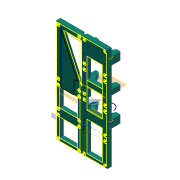
# Autodesk Inventor part: 30_CUBE_openSIM_base_v3
Saved by Autodesk Inventor 2019 (Build 230136000, 136)
## iProperties
Created: 2019-07-01
Part Number: 30_CUBE_openSIM_base_v3
Material: Generic
Document SubType Name: Modeling
Designer: diederichbenedict
Density: 1 g/cm^3
Appearance: IPHT_Türkis
Author: diederichbenedict
Autodesk Inventor part; units mm, degrees
ref_plane "YZ Plane" through (0, 0, 0) normal (1, 0, 0) x (0, 1, 0)
ref_plane "XZ Plane" through (0, 0, 0) normal (0, 1, 0) x (-1, 0, 0)
ref_plane "Work Plane1" through (181.6, 41.8, 16) normal (0, 0, -1) x (-1, 0, 0)
sketch "Sketch1" plane through (0, 41.8, 0) normal (0, 0, 1) x (1, 0, 0)
  circle A0 centre (0.9, -0.9) radius 1.45 construction
  line L0 (4, -1.5) -> (1.5, -4) construction
  line L1 (4, -1.5) -> (4, 4) construction
  line L2 (4, 4) -> (-2, 4) construction
  arc A1 (-2, 4) -> (-4, 2) centre (-2, 2) ccw construction
  line L3 (-4, 2) -> (-4, -4) construction
  line L4 (-4, -4) -> (1.5, -4) construction
  arc A2 (45.8, 2) -> (43.8, 4) centre (43.8, 2) ccw construction
  line L5 (43.8, 4) -> (37.8, 4) construction
  line L6 (37.8, 4) -> (37.8, -1.5) construction
  line L7 (40.3, -4) -> (45.8, -4) construction
  line L8 (45.8, -4) -> (45.8, 2) construction
  circle A3 centre (40.9, -0.9) radius 1.45 construction
  line L9 (37.8, -40.3) -> (40.3, -37.8) construction
  line L10 (37.8, -40.3) -> (37.8, -45.8) construction
  line L11 (37.8, -45.8) -> (43.8, -45.8) construction
  arc A4 (43.8, -45.8) -> (45.8, -43.8) centre (43.8, -43.8) ccw construction
  line L12 (45.8, -43.8) -> (45.8, -37.8) construction
  line L13 (45.8, -37.8) -> (40.3, -37.8) construction
  circle A5 centre (40.9, -40.9) radius 1.45 construction
  circle A6 centre (0.9, -40.9) radius 1.45 construction
  line L14 (1.5, -37.8) -> (4, -40.3) construction
  line L15 (1.5, -37.8) -> (-4, -37.8) construction
  line L16 (-4, -37.8) -> (-4, -43.8) construction
  arc A7 (-4, -43.8) -> (-2, -45.8) centre (-2, -43.8) ccw construction
  line L17 (-2, -45.8) -> (4, -45.8) construction
  line L18 (4, -45.8) -> (4, -40.3) construction
  line L19 (40.3, -4) -> (37.8, -1.5) construction
  line L20 (-2, 154) -> (93.8, 154)
  line L21 (95.8, 152) -> (95.8, -43.8)
  line L22 (93.8, -45.8) -> (-2, -45.8)
  line L23 (-4, -43.8) -> (-4, 152)
  line L24 (90.3, -37.8) -> (90.3, 146)
  line L25 (87.8, 148.5) -> (4, 148.5)
  line L26 (1.5, 146) -> (1.5, -37.8)
  line L27 (4, -40.3) -> (87.8, -40.3)
  line L28 (87.8, -40.3) -> (90.3, -37.8)
  line L29 (4, -40.3) -> (1.5, -37.8)
  line L30 (4, 148.5) -> (1.5, 146)
  line L31 (90.3, 146) -> (87.8, 148.5)
  arc A8 (95.8, 152) -> (93.8, 154) centre (93.8, 152) ccw
  arc A9 (93.8, -45.8) -> (95.8, -43.8) centre (93.8, -43.8) ccw
  arc A10 (-4, -43.8) -> (-2, -45.8) centre (-2, -43.8) ccw
  arc A11 (-2, 154) -> (-4, 152) centre (-2, 152) ccw
  circle A12 centre (1, -1) radius 1.4
  circle A13 centre (40.8, -1) radius 1.4
  circle A14 centre (90.8, -40.8) radius 1.4
  circle A15 centre (1, -40.8) radius 1.4
  circle A16 centre (45.9, 104.1) radius 44.4 construction
  line L32 (45.8, -37.8) -> (87.8, -37.8)
  line L33 (87.8, -37.8) -> (87.8, 146)
  line L34 (45.9, 148.5) -> (45.9, -40.3)
  line L35 (87.8, 146) -> (45.9, 146)
  line L36 (77.4, 111.7) -> (64.2, 111.7) construction
  line L37 (64.2, 96.7) -> (77.4, 96.7) construction
  line L38 (77.4, 61.7) -> (64.2, 61.7) construction
  line L39 (64.2, 46.7) -> (77.4, 46.7) construction
  line L40 (45.9, 111.7) -> (87.8, 111.7)
  line L41 (87.8, 111.7) -> (87.8, 96.7)
  line L42 (87.8, 96.7) -> (45.9, 96.7)
  line L43 (45.9, 96.7) -> (45.9, 111.7)
  line L44 (45.9, 61.7) -> (87.8, 61.7)
  line L45 (87.8, 61.7) -> (87.8, 46.7)
  line L46 (87.8, 46.7) -> (45.9, 46.7)
  line L47 (45.9, 46.7) -> (45.9, 61.7)
  point P0 (95.8, -45.8)
  point P1 (95.8, 154)
  point P2 (-4, -45.8)
  point P3 (90.3, -40.3)
  point P4 (90.3, 148.5)
  point P5 (1.5, 148.5)
  point P6 (1.5, -40.3)
  point P7 (40.8, 149)
  point P8 (45.8, -40.8)
  point P9 (45.9, -37.8)
  point P10 (63.2, 61.7)
  dimension "d34" = 99.8
  dimension "d35" = 199.8
  dimension "d36" = 5.5
  dimension "d37" = 2.5
  dimension "d38" = 2.5
  dimension "d39" = 2.5
  dimension "d40" = 2.5
  dimension "d41" = 2.5
  dimension "d42" = 2.5
  dimension "d43" = 2.5
  dimension "d44" = 2.5
  dimension "d45" = 2
  dimension "d46" = 5
  dimension "d47" = 5
  dimension "d48" = 5
  dimension "d49" = 5
  dimension "d50" = 5
  dimension "d51" = 5
  dimension "d52" = 0.5
  dimension "d53" = 5
  dimension "d54" = 5
  dimension "d55" = 2.8
  dimension "d56" = 2.8
  dimension "d57" = 2.8
  dimension "d58" = 2.8
  constraints: 48 end point, 22 point on line, 9 coincident, 9 parallel, 8 centre point, 8 point on circle, 8 tangent, 5 perpendicular, 4 horizontal, 3 equal radius, 3 midpoint, 2 vertical, 1 vertical alignment, 6 other
  measures "d34" distance of point (95.8, -45.8) point (-4, -45.8)
  measures "d35" distance of point (95.8, 154) point (95.8, -45.8)
  measures "d36" distance between parallel lines of L21 L24
  measures "d37" distance of L27.end point (90.3, -40.3)
  measures "d38" distance of L24.start point (90.3, -40.3)
  measures "d39" distance of L27.start point (1.5, -40.3)
  measures "d40" distance of L26.end point (1.5, -40.3)
  measures "d41" distance of L25.end point (1.5, 148.5)
  measures "d42" distance of L26.start point (1.5, 148.5)
  measures "d43" distance of L24.end point (90.3, 148.5)
  measures "d44" distance of L25.start point (90.3, 148.5)
  measures "d45" radius of A8
  measures "d46" distance from line of point (1, -40.8) L23
  measures "d47" distance from line of L22 point (1, -40.8)
  measures "d48" distance from line of L21 point (90.8, -40.8)
  measures "d49" distance from line of L22 point (90.8, -40.8)
  measures "d50" distance from line of L8 point (40.8, 149)
  measures "d51" distance from line of L20 point (40.8, 149)
  measures "d52" distance from line of point (1, -1) L26
  measures "d53" distance from line of L3 point (1, -1)
  measures "d54" distance from line of L2 point (1, -1)
  measures "d55" diameter of A12
  measures "d56" diameter of A13
  measures "d57" diameter of A14
  measures "d58" diameter of A15
extrude "Extrusion1" add sketch "Sketch1" along normal blind 8 contours L20 A8 L21 A9 L22 A10 L23 A11 | L28 L27 L34 L32 L33 L35 L25 L31 L24 | L27 L29 L26 A12 L30 L25 L34 | L34 L44 L33 L46 | L40 L33 L42 L34 | L26 A12 | A13 picked at (1.6831, -0.6911)
fillet "Fillet1" radius 2 8 edges at (45.9, -4, 8) (95.2142, -3.4142, 8) (95.8, 95.9, 8) (95.2142, 195.2142, 8) (45.9, 195.8, 8) (-3.4142, 195.2142, 8) (-4, 95.9, 8) (-3.4142, -3.4142, 8)
sketch "Sketch4" plane through (0, 41.8, 8) normal (0, 0, 1) x (1, 0, 0)
  circle A0 centre (1, -40.8) radius 1.4 projected
  circle A1 centre (90.8, -40.8) radius 1.4 projected
  circle A2 centre (1, -1) radius 1.4 projected
  line L0 (-2, -45.8) -> (93.8, -45.8) construction
  line L1 (4, -37.8) -> (4, 146) construction
  circle A3 centre (1, -40.8) radius 1.4 construction
  circle A4 centre (1, -40.8) radius 1.4 construction
  circle A5 centre (1, -1) radius 1.4
  circle A6 centre (1, -40.8) radius 1.4
  line L2 (1, -1) -> (41, -1) construction
  line L3 (41, -1) -> (41, -41) construction
  line L4 (41, -41) -> (1, -41) construction
  line L5 (1, -41) -> (1, -1) construction
  circle A7 centre (1, 9.2) radius 1.4 construction
  circle A8 centre (1, 49) radius 1.4
  circle A9 centre (1, 9.2) radius 1.4
  line L6 (1, 49) -> (41, 49) construction
  line L7 (41, 49) -> (41, 9) construction
  line L8 (41, 9) -> (1, 9) construction
  line L9 (1, 9) -> (1, 49) construction
  circle A10 centre (1, 59.2) radius 1.4 construction
  circle A11 centre (1, 99) radius 1.4
  circle A12 centre (1, 59.2) radius 1.4
  line L10 (1, 99) -> (41, 99) construction
  line L11 (41, 99) -> (41, 59) construction
  line L12 (41, 59) -> (1, 59) construction
  line L13 (1, 59) -> (1, 99) construction
  circle A13 centre (1, 109.2) radius 1.4 construction
  circle A14 centre (1, 149) radius 1.4
  circle A15 centre (1, 109.2) radius 1.4
  line L14 (1, 149) -> (41, 149) construction
  line L15 (41, 149) -> (41, 109) construction
  line L16 (41, 109) -> (1, 109) construction
  line L17 (1, 109) -> (1, 149) construction
  circle A16 centre (51, -40.8) radius 1.4 construction
  circle A17 centre (51, -1) radius 1.4
  circle A18 centre (51, -40.8) radius 1.4
  line L18 (51, -1) -> (91, -1) construction
  line L19 (91, -1) -> (91, -41) construction
  line L20 (91, -41) -> (51, -41) construction
  line L21 (51, -41) -> (51, -1) construction
  circle A19 centre (51, 9.2) radius 1.4 construction
  circle A20 centre (51, 49) radius 1.4
  circle A21 centre (51, 9.2) radius 1.4
  line L22 (51, 49) -> (91, 49) construction
  line L23 (91, 49) -> (91, 9) construction
  line L24 (91, 9) -> (51, 9) construction
  line L25 (51, 9) -> (51, 49) construction
  circle A22 centre (51, 59.2) radius 1.4 construction
  circle A23 centre (51, 99) radius 1.4
  circle A24 centre (51, 59.2) radius 1.4
  line L26 (51, 99) -> (91, 99) construction
  line L27 (91, 99) -> (91, 59) construction
  line L28 (91, 59) -> (51, 59) construction
  line L29 (51, 59) -> (51, 99) construction
  circle A25 centre (51, 109.2) radius 1.4 construction
  circle A26 centre (51, 149) radius 1.4
  circle A27 centre (51, 109.2) radius 1.4
  line L30 (51, 149) -> (91, 149) construction
  line L31 (91, 149) -> (91, 109) construction
  line L32 (91, 109) -> (51, 109) construction
  line L33 (51, 109) -> (51, 149) construction
  point P0 (-2, 4.2)
  point P1 (4, 12.2)
  point P2 (-2, 54.2)
  point P3 (4, 62.2)
  point P4 (-2, 104.2)
  point P5 (4, 112.2)
  point P6 (48, -45.8)
  point P7 (54, -37.8)
  point P8 (48, 4.2)
  point P9 (54, 12.2)
  point P10 (48, 54.2)
  point P11 (54, 62.2)
  point P12 (48, 104.2)
  point P13 (54, 112.2)
  dimension "d106" = 40
  dimension "d107" = 40
  dimension "d110" = 50
  dimension "d113" = 50
  constraints: 64 end point, 24 centre point, 24 coincident, 3 concentric, 2 horizontal, 2 parallel, 1 perpendicular, 1 vertical, 140 other
  measures "d106" distance of L3.end L4.end
  measures "d107" distance of L2.end L3.end
  measures "d110" distance of A0.centre point (1, 9.2)
  measures "d113" distance of A0.centre point (51, -40.8)
hole "Hole2" at (1, 40.8, 8) at (1, 1, 8) at (90.8, 1, 8) at (91, 190.8, 8) at (91, 150.8, 8) at (91, 140.8, 8) at (91, 100.8, 8) at (91, 90.8, 8) at (91, 50.8, 8) at (91, 40.8, 8) at (51, 0.8, 8) at (41, 0.8, 8) at (1, 50.8, 8) at (1, 90.8, 8) at (1, 100.8, 8) at (1, 190.8, 8) at (41, 190.8, 8) at (51, 190.8, 8) at (41, 90.8, 8) at (41, 100.8, 8) at (41, 140.8, 8) at (41, 150.8, 8) at (41, 50.8, 8) at (41, 40.8, 8) at (51, 101, 8) at (51, 90.8, 8) at (51, 140.8, 8) at (51, 151, 8) direction (0, 0, -1) diameter 3.2 depth 12 tip angle 118 counterbore diameter 6 counterbore depth 2.5
sketch "Sketch23" plane through (0, 41.8, 0) normal (0, 0, -1) x (-1, 0, 0)
  circle A0 centre (-41, 149) radius 1.6 projected
  circle A1 centre (-1, 59) radius 1.6 projected
  circle A2 centre (-1, 9) radius 1.6 projected
  circle A3 centre (-51, -41) radius 1.6 projected
  circle A4 centre (-91, 9) radius 1.6 projected
  circle A5 centre (-91, 59) radius 1.6 projected
  circle A6 centre (-91, 109) radius 1.6 projected
  circle A7 centre (-90.8, -40.8) radius 1.6 projected
  circle A8 centre (-1, -1) radius 1.6 projected
  circle A9 centre (-1, -40.8) radius 1.6 projected
  circle A10 centre (-91, 149) radius 1.6 projected
  circle A11 centre (-91, 99) radius 1.6 projected
  circle A12 centre (-91, 49) radius 1.6 projected
  circle A13 centre (-91, -1) radius 1.6 projected
  circle A14 centre (-41, -41) radius 1.6 projected
  circle A15 centre (-1, 49) radius 1.6 projected
  circle A16 centre (-1, 149) radius 1.6 projected
  circle A17 centre (-51, 149) radius 1.6 projected
  line L0 (-87.8, 111.7) -> (-45.9, 111.7) projected
  line L1 (-87.8, 111.7) -> (-87.8, 146) projected
  line L2 (-87.8, 146) -> (-45.9, 146) projected
  line L3 (-45.9, 146) -> (-45.9, 111.7) projected
  line L4 (-45.9, 96.7) -> (-45.9, 61.7) projected
  line L5 (-87.8, 61.7) -> (-45.9, 61.7) projected
  line L6 (-87.8, 61.7) -> (-87.8, 96.7) projected
  line L7 (-45.9, 96.7) -> (-87.8, 96.7) projected
  line L8 (-45.9, -37.8) -> (-87.8, -37.8) projected
  line L9 (-87.8, -37.8) -> (-87.8, 46.7) projected
  line L10 (-45.9, 46.7) -> (-87.8, 46.7) projected
  line L11 (-45.9, 46.7) -> (-45.9, -37.8) projected
  line L12 (-95.8, 152) -> (-95.8, -43.8) projected
  arc A18 (-95.8, -43.8) -> (-93.8, -45.8) centre (-93.8, -43.8) ccw projected
  line L13 (-93.8, -45.8) -> (2, -45.8) projected
  arc A19 (2, -45.8) -> (4, -43.8) centre (2, -43.8) ccw projected
  line L14 (4, -43.8) -> (4, 152) projected
  arc A20 (4, 152) -> (2, 154) centre (2, 152) ccw projected
  line L15 (2, 154) -> (-93.8, 154) projected
  arc A21 (-93.8, 154) -> (-95.8, 152) centre (-93.8, 152) ccw projected
  point P0 (0, -41.8)
extrude "Extrusion15" add sketch "Sketch23" against normal up to surface (8 mm away) contours L1 L2 L3 L0 | L4 L5 L6 L7 | L8 L9 L10 L11
ref_plane "Work Plane5" through (-11.0179, 119.2166, -1.971) normal (0, 0, 1) x (0.9026, 0.4305, 0)
sketch "Sketch26" plane through (0, 41.8, 0) normal (0, 0, 1) x (1, 0, 0)
  arc A0 (7.0096, 100.7998) -> (7.6791, 99.3501) centre (6.3003, 99.5928) ccw construction
  line L0 (19.4325, 78.671) -> (-0.7895, 122.4569) construction
  circle A1 centre (21.0984, 106.427) radius 1.4 construction
  line L1 (10.8532, 105.175) -> (33.6761, 57.3258) construction
  circle A2 centre (33.6761, 57.3258) radius 2.1706
  circle A3 centre (3.6505, 101.3448) radius 1.4
  arc A4 (19.4922, 109.1893) -> (19.7163, 108.7194) centre (18.3626, 108.3621) ccw
  line L2 (18.3626, 108.3621) -> (3.6505, 101.3448)
  line L3 (11.0066, 104.8535) -> (33.6998, 57.2762)
  line L4 (18.3626, 108.3621) -> (3.6505, 101.3448) construction
  line L5 (3.6505, 101.3448) -> (0.9579, 106.9899) construction
  line L6 (0.9579, 106.9899) -> (15.67, 114.0073) construction
  line L7 (15.67, 114.0073) -> (18.3626, 108.3621) construction
  line L8 (18.3626, 108.3621) -> (3.6505, 101.3448) construction
  line L9 (3.6505, 101.3448) -> (7.9556, 92.319) construction
  line L10 (7.9556, 92.319) -> (22.6677, 99.3363) construction
  line L11 (22.6677, 99.3363) -> (18.3626, 108.3621) construction
  point P0 (0, -41.8)
  point P1 (3.5305, 101.5964)
  point P2 (18.2427, 108.6137)
  point P3 (18.2427, 108.6137)
  dimension "d266" = 90
  dimension "d267" = 8.15
  dimension "d268" = 10
  constraints: 22 end point, 5 equal length, 3 centre point, 2 coincident, 2 perpendicular, 2 point on circle, 1 midpoint, 1 point on line, 8 other
  measures "d266" angle of L2 L3
  measures "d267" distance from line of L2.start L3
  measures "d268" distance of L9.end L2.end
ref_plane "Work Plane6" through (-2, 180.8, 0) normal (0, 1, 0) x (1, 0, 0)
sketch "Sketch27" plane through (-2, 180.8, 0) normal (0, 1, 0) x (1, 0, 0)
  circle A0 centre (72.821, 16.921) radius 15.24 construction
  circle A1 centre (72.821, 16.921) radius 14.99 construction
  line L0 (72.821, 16.921) -> (88.9923, 33.0923) construction
  line L1 (72.821, 16.921) -> (95.6907, 16.921) construction
  line L2 (57.831, 16.921) -> (72.3888, 19.4879) construction
  line L3 (57.831, 16.921) -> (49.8, 16.921) construction
  line L4 (49.8, 16.921) -> (49.8, 0)
  line L5 (0, 0) -> (95.8, 0) projected
  line L6 (97.8, 28.4358) -> (97.8, 0)
  line L7 (49.8, 16.921) -> (55.8, 16.921)
  line L8 (55.8, 16.921) -> (63.6642, 1.1093)
  line L9 (95.8, 0) -> (0, 0) projected
  line L10 (97.8, 16.921) -> (89.842, 16.921)
  line L11 (89.842, 16.921) -> (81.9776, 1.1093)
  line L12 (65.455, 0) -> (80.1869, 0)
  arc A2 (63.6642, 1.1093) -> (65.455, 0) centre (65.455, 2) ccw
  arc A3 (80.1869, 0) -> (81.9776, 1.1093) centre (80.1869, 2) ccw
  line L13 (97.8, 0) -> (95.8, 0) projected
  line L14 (97.8, 0) -> (80.1869, 0)
  line L15 (65.455, 0) -> (49.8, 0)
  point P0 (2, 0)
  point P1 (62.2214, 6.3214)
  point P2 (83.4205, 27.5205)
  point P3 (64.216, 0)
  point P4 (81.4259, 0)
  dimension "d180" = 0.25
  dimension "d181" = 45
  dimension "d182" = 145
  dimension "d240" = 48
  dimension "d242" = 17.021
  dimension "d243" = 2
  dimension "d244" = 26.445
  constraints: 26 end point, 14 point on line, 8 point on circle, 7 tangent, 4 centre point, 4 collinear, 2 horizontal, 1 coincident, 1 equal length, 1 equal radius, 1 perpendicular, 2 other
  measures "d180" radial gap between concentric circles of A0 A1
  measures "d181" angle of L1 L0
  measures "d182" angle of L0 L2
  measures "d240" distance between parallel lines of L6 L4
  measures "d242" distance of L10.end L0.start
  measures "d243" radius of A2
  measures "d244" angle of L6 L11
extrude "Extrusion17" add sketch "Sketch27" against normal blind 15
ref_plane "Work Plane7" through (-2, 75.8, 0) normal (0, 1, 0) x (1, 0, 0)
sketch "Sketch28" plane through (-2, 75.8, 0) normal (0, 1, 0) x (1, 0, 0)
  line L0 (49.8, 16.921) -> (49.8, 0) projected
  line L1 (65.455, 0) -> (49.8, 0) projected
  arc A0 (63.6642, 1.1093) -> (65.455, 0) centre (65.455, 2) ccw projected
  line L2 (63.6642, 1.1093) -> (55.8, 16.921) projected
  line L3 (55.8, 16.921) -> (49.8, 16.921) projected
  line L4 (97.8, 0) -> (97.8, 16.921) projected
  line L5 (97.8, 16.921) -> (89.842, 16.921) projected
  line L6 (89.842, 16.921) -> (81.9776, 1.1093) projected
  arc A1 (80.1869, 0) -> (81.9776, 1.1093) centre (80.1869, 2) ccw projected
  line L7 (97.8, 0) -> (80.1869, 0) projected
  line L8 (97.8, 16.921) -> (97.8, 0) projected
  line L9 (80.1869, 0) -> (97.8, 0) projected
  arc A2 (80.1869, 0) -> (81.9776, 1.1093) centre (80.1869, 2) ccw projected
  line L10 (81.9776, 1.1093) -> (89.842, 16.921) projected
  line L11 (89.842, 16.921) -> (97.8, 16.921) projected
  point P0 (2, 0)
extrude "Extrusion18" add sketch "Sketch28" against normal blind 15
sketch "Sketch29" plane through (0, 41.8, 8) normal (0, 0, 1) x (1, 0, 0)
  point P0 (0, -41.8)
sketch "Sketch30" plane through (0, 41.8, 0) normal (0, 0, -1) x (-1, 0, 0)
  line L0 (-63.455, 34) -> (-47.8, 34) projected
  line L1 (-47.8, 19) -> (-63.455, 19) projected
  circle A0 centre (-91, 109) radius 1.6 projected
  arc A1 (4, 152) -> (2, 154) centre (2, 152) ccw projected
  line L2 (2, 154) -> (-93.8, 154) projected
  arc A2 (-93.8, 154) -> (-95.8, 152) centre (-93.8, 152) ccw projected
  line L3 (-95.8, 152) -> (-95.8, 139) projected
  arc A3 (-95.8, -43.8) -> (-93.8, -45.8) centre (-93.8, -43.8) ccw projected
  line L4 (-93.8, -45.8) -> (2, -45.8) projected
  arc A4 (2, -45.8) -> (4, -43.8) centre (2, -43.8) ccw projected
  circle A5 centre (-41, 149) radius 1.6 projected
  circle A6 centre (-1, 59) radius 1.6 projected
  circle A7 centre (-1, 9) radius 1.6 projected
  circle A8 centre (-51, -41) radius 1.6 projected
  circle A9 centre (-91, 9) radius 1.6 projected
  circle A10 centre (-91, 59) radius 1.6 projected
  circle A11 centre (-90.8, -40.8) radius 1.6 projected
  circle A12 centre (-1, -1) radius 1.6 projected
  circle A13 centre (-1, -40.8) radius 1.6 projected
  circle A14 centre (-91, 149) radius 1.6 projected
  circle A15 centre (-91, 99) radius 1.6 projected
  circle A16 centre (-91, 49) radius 1.6 projected
  circle A17 centre (-91, -1) radius 1.6 projected
  circle A18 centre (-41, -41) radius 1.6 projected
  circle A19 centre (-1, 49) radius 1.6 projected
  circle A20 centre (-1, 149) radius 1.6 projected
  circle A21 centre (-51, 149) radius 1.6 projected
  line L5 (6.5, -43.3) -> (-43.3, -43.3) construction
  line L6 (-43.3, -43.3) -> (-43.3, 6.5) construction
  line L7 (-43.3, 6.5) -> (6.5, 6.5) construction
  line L8 (6.5, 6.5) -> (6.5, -43.3) construction
  line L9 (-93.3, -43.3) -> (-43.5, -43.3) construction
  line L10 (-43.5, -43.3) -> (-43.5, 6.5) construction
  line L11 (-43.5, 6.5) -> (-93.3, 6.5) construction
  line L12 (-93.3, 6.5) -> (-93.3, -43.3) construction
  line L13 (-56.9142, 124) -> (-85.811, 124) construction
  line L14 (-81.9373, 124) -> (-81.9373, 139) construction
  line L15 (-56.9142, 124) -> (-81.9373, 124) construction
  line L16 (-56.9142, 139) -> (-56.9142, 124) construction
  line L17 (-56.9142, 139) -> (-81.9373, 139) construction
  circle A22 centre (-69.55, -19.75) radius 26.25 construction
  line L18 (-38.4, -38.5) -> (-3.4, -38.5) construction
  line L19 (-3.4, -38.5) -> (-3.4, -3.5) construction
  line L20 (-3.4, -3.5) -> (-38.4, -3.5) construction
  line L21 (-38.4, -3.5) -> (-38.4, -38.5) construction
  line L22 (-38.4, -38.5) -> (-3.4, -3.5) construction
  line L23 (-3.4, -38.5) -> (-38.4, -3.5) construction
  line L24 (-38.4, -3.5) -> (-3.4, -3.5)
  line L25 (-3.4, -3.5) -> (-3.4, -38.5)
  line L26 (-3.4, -38.5) -> (-38.4, -38.5)
  line L27 (-38.4, -38.5) -> (-38.4, -3.5)
  line L28 (-38.4, -3.5) -> (-3.4, -38.5) construction
  line L29 (-3.4, -3.5) -> (-38.4, -38.5) construction
  line L30 (6.5, 6.5) -> (-43.3, 6.5)
  line L31 (-43.3, 6.5) -> (-43.3, 56.3)
  line L32 (-43.3, 56.3) -> (6.5, 56.3)
  line L33 (6.5, 56.3) -> (6.5, 6.5) construction
  line L34 (-3.4, 46.3229) -> (-38.4, 46.3229)
  line L35 (-38.4, 46.3229) -> (-38.4, 11.3229)
  line L36 (-38.4, 11.3229) -> (-3.4, 11.3229)
  line L37 (-3.4, 11.3229) -> (-3.4, 46.3229)
  line L38 (-3.4, 46.3229) -> (-38.4, 11.3229) construction
  line L39 (-38.4, 46.3229) -> (-3.4, 11.3229) construction
  line L40 (-55.8, -38.5) -> (-85.8, -38.5)
  line L41 (-85.8, -38.5) -> (-85.8, 6.5)
  line L42 (-85.8, 6.5) -> (-55.8, 6.5)
  line L43 (-55.8, 6.5) -> (-55.8, -38.5)
  line L44 (-7.9405, 76.5555) -> (-34.9278, 89.4278) projected
  line L45 (-10.9392, 144.6427) -> (-45.9, 144.6427)
  line L46 (-45.9, 144.6427) -> (-45.9, 71.4872)
  line L47 (-63.455, 34) -> (-78.1869, 34) projected
  line L48 (-55.8, 124) -> (-85.8, 124)
  line L49 (-85.8, 124) -> (-85.8, 34)
  line L50 (-85.8, 34) -> (-55.8, 34)
  line L51 (-55.8, 34) -> (-55.8, 124)
  line L52 (-78.1869, 19) -> (-63.455, 19) projected
  line L53 (-55.8, 6.5) -> (-85.8, 6.5)
  line L54 (-85.8, 6.5) -> (-85.8, 19)
  line L55 (-85.8, 19) -> (-55.8, 19)
  line L56 (-55.8, 19) -> (-55.8, 6.5)
  circle A23 centre (-51, 109.2) radius 1.6 projected
  line L57 (-10.9392, 144.6427) -> (-45.9, 68.723)
  line L58 (-45.9, 68.723) -> (-45.9, 71.4872)
  line L59 (4, -43.8) -> (4, 152) projected
  line L60 (-63.455, 19) -> (-63.455, 34) projected
  line L61 (-95.8, 139) -> (-78.1869, 139) projected
  line L62 (-78.1869, 124) -> (-78.1869, 139) projected
  line L63 (-78.1869, 124) -> (-95.8, 124) projected
  line L64 (-95.8, 124) -> (-95.8, 34) projected
  line L65 (-95.8, 34) -> (-78.1869, 34) projected
  line L66 (-78.1869, 19) -> (-78.1869, 34) projected
  line L67 (-78.1869, 19) -> (-95.8, 19) projected
  line L68 (-95.8, 19) -> (-95.8, -43.8) projected
  line L69 (-47.8, 34) -> (-47.8, 19) projected
  line L70 (-1, 9) -> (-41.0771, 49) construction
  point P0 (0, -41.8)
  point P1 (-90.5546, 19)
  point P2 (-90.5546, 34)
  point P3 (-45.8, 34)
  point P4 (-45.8, 19)
  point P5 (-20.9, -21)
  point P6 (-20.9, -21)
  dimension "d191" = 49.8
  dimension "d192" = 49.8
  dimension "d193" = 49.8
  dimension "d194" = 49.8
  dimension "d196" = 35
  dimension "d197" = 35
  dimension "d198" = 49.8
  dimension "d199" = 35
  dimension "d200" = 35
  dimension "d205" = 45
  constraints: 94 end point, 18 parallel, 10 horizontal, 10 perpendicular, 5 midpoint, 4 point on line, 3 tangent, 1 centre point, 1 collinear, 1 vertical
  measures "d191" distance of L6.end L7.end
  measures "d192" distance of L5.end L6.end
  measures "d193" distance of L11.end L10.end
  measures "d194" distance of L10.end L9.end
  measures "d196" distance of L20.end L19.end
  measures "d197" distance of L19.end L18.end
  measures "d198" distance of L30.end L31.end
  measures "d199" distance of L36.end L35.end
  measures "d200" distance of L35.end L34.end
  measures "d205" distance of L40.end L41.end
extrude "Extrusion19" cut sketch "Sketch30" against normal blind 15 contours L47 L50 L49 L48 L51 L0 | L1 L56 L42 L54 L55 L52 | L43 L40 L41 L42 | L24 L25 L26 L27 | L37 L36 L35 L34 | L57 L58 L46 L45
sketch "Sketch31" plane through (-2, 180.8, 0) normal (0, 1, 0) x (1, 0, 0)
  circle A0 centre (47.8, -1.2) radius 3.1
  line L0 (97.8, -1.7) -> (97.8, -4.5) projected
  line L1 (95.8, 0) -> (0, 0) projected
  point P0 (2, 0)
  dimension "d207" = 6.2
  dimension "d208" = 50
  dimension "d209" = 1.2
  constraints: 1 centre point
  measures "d207" diameter of A0
  measures "d208" distance from line of A0.centre L0
  measures "d209" distance from line of A0.centre L1
extrude "Extrusion20" cut sketch "Sketch31" along normal through all both and the other way through all
sketch "Sketch34" plane through (0, 41.8, 8) normal (0, 0, 1) x (1, 0, 0)
  line L0 (85.8, 124) -> (85.8, 34) projected
  line L1 (85.8, 34) -> (55.8, 34) projected
  line L2 (85.8, -38.5) -> (55.8, -38.5) projected
  line L3 (55.8, -38.5) -> (55.8, 19) projected
  line L4 (55.8, 19) -> (85.8, 19) projected
  line L5 (85.8, 19) -> (85.8, -38.5) projected
  line L6 (3.4, -3.5) -> (38.4, -3.5) projected
  line L7 (38.4, -3.5) -> (38.4, -38.5) projected
  line L8 (38.4, -38.5) -> (3.4, -38.5) projected
  line L9 (3.4, -38.5) -> (3.4, -3.5) projected
  line L10 (10.9392, 144.6427) -> (45.9, 144.6427) projected
  line L11 (45.9, 144.6427) -> (45.9, 68.723) projected
  line L12 (38.4, 46.3229) -> (38.4, 11.3229) projected
  line L13 (38.4, 11.3229) -> (3.4, 11.3229) projected
  line L14 (3.4, 11.3229) -> (3.4, 46.3229) projected
  line L15 (3.4, 46.3229) -> (38.4, 46.3229) projected
  line L16 (-2, -43.8) -> (-2, -40.8) projected
  circle A0 centre (1, 59) radius 3 projected
  line L17 (-2, 49) -> (-2, 59) projected
  circle A1 centre (1, 49) radius 3 projected
  line L18 (-2, 9) -> (-2, 49) projected
  circle A2 centre (1, 9) radius 3 projected
  line L19 (-2, -1) -> (-2, 9) projected
  circle A3 centre (1, -1) radius 3 projected
  line L20 (-2, -40.8) -> (-2, -1) projected
  arc A4 (1, -43.8) -> (-2, -40.8) centre (1, -40.8) ccw projected
  line L21 (39.923, -43.8) -> (1, -43.8) projected
  arc A5 (42.077, -43.8) -> (39.923, -43.8) centre (41, -41) ccw projected
  line L22 (49.923, -43.8) -> (42.077, -43.8) projected
  arc A6 (52.077, -43.8) -> (49.923, -43.8) centre (51, -41) ccw projected
  line L23 (90.8, -43.8) -> (52.077, -43.8) projected
  arc A7 (93.8, -40.8) -> (90.8, -43.8) centre (90.8, -40.8) ccw projected
  line L24 (93.8, -2.077) -> (93.8, -40.8) projected
  arc A8 (93.8, 0.077) -> (93.8, -2.077) centre (91, -1) ccw projected
  line L25 (93.8, 7.923) -> (93.8, 0.077) projected
  arc A9 (93.8, 10.077) -> (93.8, 7.923) centre (91, 9) ccw projected
  line L26 (93.8, 47.923) -> (93.8, 10.077) projected
  arc A10 (93.8, 50.077) -> (93.8, 47.923) centre (91, 49) ccw projected
  line L27 (93.8, 57.923) -> (93.8, 50.077) projected
  arc A11 (93.8, 60.077) -> (93.8, 57.923) centre (91, 59) ccw projected
  line L28 (93.8, 97.923) -> (93.8, 60.077) projected
  arc A12 (93.8, 100.077) -> (93.8, 97.923) centre (91, 99) ccw projected
  line L29 (93.8, 107.923) -> (93.8, 100.077) projected
  arc A13 (93.8, 110.077) -> (93.8, 107.923) centre (91, 109) ccw projected
  line L30 (93.8, 147.923) -> (93.8, 110.077) projected
  arc A14 (91, 152) -> (93.8, 147.923) centre (91, 149) ccw projected
  line L31 (51, 152) -> (91, 152) projected
  circle A15 centre (51, 149) radius 3 projected
  line L32 (41, 152) -> (51, 152) projected
  circle A16 centre (41, 149) radius 3 projected
  line L33 (1, 152) -> (41, 152) projected
  arc A17 (-2, 149) -> (1, 152) centre (1, 149) ccw projected
  line L34 (-2, 59) -> (-2, 149) projected
  line L35 (-2, 149) -> (-2, 152) projected
  arc A18 (49.3417, 61.7) -> (52.6583, 61.7) centre (51, 59.2) ccw projected
  line L36 (52.6583, 61.7) -> (49.3417, 61.7) projected
  arc A19 (49.3417, 111.7) -> (52.6583, 111.7) centre (51, 109.2) ccw projected
  line L37 (52.6583, 111.7) -> (49.3417, 111.7) projected
  line L38 (49.0739, 46.7) -> (52.9261, 46.7) projected
  arc A20 (52.9261, 46.7) -> (49.0739, 46.7) centre (51, 49) ccw projected
  circle A21 centre (41, -1) radius 3 projected
  circle A22 centre (41, 59) radius 3 projected
  circle A23 centre (41, 49) radius 3 projected
  circle A24 centre (41, 9) radius 3 projected
  line L39 (49.0739, 96.7) -> (52.9261, 96.7) projected
  arc A25 (52.9261, 96.7) -> (49.0739, 96.7) centre (51, 99) ccw projected
  line L40 (9.6212, 135.0512) -> (38, 72.8149)
  line L41 (38, 72.8149) -> (30.9112, 72.8149)
  line L42 (42.7, -45.8) -> (42.7, 154) projected
  line L43 (30.9112, 72.8149) -> (30.9112, 46.7)
  line L44 (30.9112, 46.7) -> (5.9734, 46.7)
  line L45 (5.9734, 46.7) -> (5.9734, 143.0509)
  line L46 (5.9734, 143.0509) -> (9.6212, 135.0512)
  line L47 (55.8, 34) -> (55.8, 124) projected
  line L48 (45.9, 68.723) -> (10.9392, 144.6427) projected
  line L49 (55.8, 124) -> (85.8, 124) projected
  arc A26 (-2, -40.8) -> (1, -43.8) centre (1, -40.8) ccw projected
  line L50 (1, -43.8) -> (-2, -43.8) projected
  arc A27 (1, 152) -> (-2, 149) centre (1, 149) ccw projected
  line L51 (-2, 152) -> (1, 152) projected
  point P0 (0, -41.8)
  constraints: 12 end point, 4 horizontal alignment, 4 perpendicular, 2 vertical alignment, 1 collinear, 1 point on line
ref_plane "Work Plane8" through (-2, 115.8, 0) normal (0, 1, 0) x (1, 0, 0)
sketch "Sketch35" plane through (-2, 115.8, 0) normal (0, 1, 0) x (1, 0, 0)
  line L0 (49.8, 16.921) -> (49.8, 1.1685) projected
  line L1 (57.8, 0) -> (50.6583, 0) projected
  line L2 (57.8, 0) -> (57.8, -8) projected
  line L3 (87.8, -8) -> (57.8, -8) projected
  line L4 (87.8, 0) -> (87.8, -8) projected
  line L5 (97.8, 0) -> (87.8, 0) projected
  arc A0 (50.6583, 0) -> (49.8, 1.1685) centre (47.8, -1.2) ccw projected
  arc A1 (63.6642, 1.1093) -> (65.455, 0) centre (65.455, 2) ccw projected
  line L6 (63.6642, 1.1093) -> (55.8, 16.921) projected
  line L7 (55.8, 16.921) -> (49.8, 16.921) projected
  arc A2 (50.6583, 0) -> (49.8, 1.1685) centre (47.8, -1.2) ccw projected
  line L8 (49.8, 1.1685) -> (49.8, 16.921) projected
  line L9 (49.8, 16.921) -> (55.8, 16.921) projected
  line L10 (55.8, 16.921) -> (63.6642, 1.1093) projected
  arc A3 (63.6642, 1.1093) -> (65.455, 0) centre (65.455, 2) ccw projected
  line L11 (80.1869, 0) -> (65.455, 0) projected
  arc A4 (80.1869, 0) -> (81.9776, 1.1093) centre (80.1869, 2) ccw projected
  line L12 (81.9776, 1.1093) -> (89.842, 16.921) projected
  line L13 (89.842, 16.921) -> (97.8, 16.921) projected
  line L14 (97.8, 16.921) -> (97.8, 0) projected
  line L15 (87.8, 0) -> (97.8, 0) projected
  line L16 (87.8, 0) -> (87.8, -8) projected
  line L17 (57.8, -8) -> (87.8, -8) projected
  line L18 (57.8, 0) -> (57.8, -8) projected
  line L19 (50.6583, 0) -> (57.8, 0) projected
  line L20 (97.8, 0) -> (97.8, 16.921) projected
  line L21 (97.8, 16.921) -> (89.842, 16.921) projected
  line L22 (89.842, 16.921) -> (81.9776, 1.1093) projected
  arc A5 (80.1869, 0) -> (81.9776, 1.1093) centre (80.1869, 2) ccw projected
  line L23 (65.455, 0) -> (80.1869, 0) projected
  point P0 (2, 0)
extrude "Extrusion22" add sketch "Sketch35" along normal blind 10
sketch "Sketch36" plane through (0, 41.8, 8) normal (0, 0, 1) x (1, 0, 0)
  line L0 (85.8, 74) -> (85.8, 34) construction
  line L1 (85.8, 34) -> (55.8, 34) construction
  line L2 (55.8, 34) -> (55.8, 74) construction
  line L3 (55.8, 84) -> (55.8, 124) construction
  line L4 (85.8, 124) -> (85.8, 84) construction
  line L5 (85.8, -38.5) -> (55.8, -38.5) construction
  line L6 (55.8, -38.5) -> (55.8, 19) construction
  line L7 (55.8, 19) -> (85.8, 19) construction
  line L8 (85.8, 19) -> (85.8, -38.5) construction
  line L9 (3.4, -3.5) -> (38.4, -3.5) construction
  line L10 (38.4, -3.5) -> (38.4, -38.5) construction
  line L11 (38.4, -38.5) -> (3.4, -38.5) construction
  line L12 (3.4, -38.5) -> (3.4, -3.5) construction
  line L13 (10.9392, 144.6427) -> (45.9, 144.6427) construction
  line L14 (45.9, 144.6427) -> (45.9, 68.723) construction
  line L15 (38.4, 46.3229) -> (38.4, 11.3229) construction
  line L16 (38.4, 11.3229) -> (3.4, 11.3229) construction
  line L17 (3.4, 11.3229) -> (3.4, 46.3229) construction
  line L18 (3.4, 46.3229) -> (38.4, 46.3229) construction
  line L19 (-2, -43.8) -> (-2, -40.8) construction
  circle A0 centre (1, 59) radius 3 construction
  line L20 (-2, 49) -> (-2, 59) construction
  circle A1 centre (1, 49) radius 3 construction
  line L21 (-2, 9) -> (-2, 49) construction
  circle A2 centre (1, 9) radius 3 construction
  line L22 (-2, -1) -> (-2, 9) construction
  circle A3 centre (1, -1) radius 3 construction
  line L23 (-2, -40.8) -> (-2, -1) construction
  arc A4 (1, -43.8) -> (-2, -40.8) centre (1, -40.8) ccw construction
  line L24 (39.923, -43.8) -> (1, -43.8) construction
  arc A5 (42.077, -43.8) -> (39.923, -43.8) centre (41, -41) ccw construction
  line L25 (49.923, -43.8) -> (42.077, -43.8) construction
  arc A6 (52.077, -43.8) -> (49.923, -43.8) centre (51, -41) ccw construction
  line L26 (90.8, -43.8) -> (52.077, -43.8) construction
  arc A7 (93.8, -40.8) -> (90.8, -43.8) centre (90.8, -40.8) ccw construction
  line L27 (93.8, -2.077) -> (93.8, -40.8) construction
  arc A8 (93.8, 0.077) -> (93.8, -2.077) centre (91, -1) ccw construction
  line L28 (93.8, 7.923) -> (93.8, 0.077) construction
  arc A9 (93.8, 10.077) -> (93.8, 7.923) centre (91, 9) ccw construction
  line L29 (93.8, 47.923) -> (93.8, 10.077) construction
  arc A10 (93.8, 50.077) -> (93.8, 47.923) centre (91, 49) ccw construction
  line L30 (93.8, 57.923) -> (93.8, 50.077) construction
  arc A11 (93.8, 60.077) -> (93.8, 57.923) centre (91, 59) ccw construction
  line L31 (93.8, 97.923) -> (93.8, 60.077) construction
  arc A12 (93.8, 100.077) -> (93.8, 97.923) centre (91, 99) ccw construction
  line L32 (93.8, 107.923) -> (93.8, 100.077) construction
  arc A13 (93.8, 110.077) -> (93.8, 107.923) centre (91, 109) ccw construction
  line L33 (93.8, 147.923) -> (93.8, 110.077) construction
  arc A14 (91, 152) -> (93.8, 147.923) centre (91, 149) ccw construction
  line L34 (51, 152) -> (91, 152) construction
  circle A15 centre (51, 149) radius 3 construction
  line L35 (41, 152) -> (51, 152) construction
  circle A16 centre (41, 149) radius 3 construction
  line L36 (1, 152) -> (41, 152) construction
  arc A17 (-2, 149) -> (1, 152) centre (1, 149) ccw construction
  line L37 (-2, 59) -> (-2, 149) construction
  line L38 (-2, 149) -> (-2, 152) construction
  arc A18 (49.3417, 61.7) -> (52.6583, 61.7) centre (51, 59.2) ccw construction
  line L39 (52.6583, 61.7) -> (49.3417, 61.7) construction
  arc A19 (49.3417, 111.7) -> (52.6583, 111.7) centre (51, 109.2) ccw construction
  line L40 (52.6583, 111.7) -> (49.3417, 111.7) construction
  line L41 (49.0739, 46.7) -> (52.9261, 46.7) construction
  arc A20 (52.9261, 46.7) -> (49.0739, 46.7) centre (51, 49) ccw construction
  circle A21 centre (41, -1) radius 3 construction
  circle A22 centre (41, 59) radius 3 construction
  circle A23 centre (41, 49) radius 3 construction
  circle A24 centre (41, 9) radius 3 construction
  line L42 (49.0739, 96.7) -> (52.9261, 96.7) construction
  arc A25 (52.9261, 96.7) -> (49.0739, 96.7) centre (51, 99) ccw construction
  line L43 (90.8, -40.8) -> (51, -40.8) construction
  line L44 (51, -40.8) -> (51, -1) construction
  line L45 (51, -1) -> (90.8, -1) construction
  line L46 (90.8, -1) -> (90.8, -40.8) construction
  line L47 (91, 9) -> (51, 9) construction
  line L48 (51, 9) -> (51, 49) construction
  line L49 (51, 49) -> (91, 49) construction
  line L50 (91, 49) -> (91, 9) construction
  line L51 (91, 59) -> (51, 59) construction
  line L52 (51, 59) -> (51, 99) construction
  line L53 (51, 99) -> (91, 99) construction
  line L54 (91, 99) -> (91, 59) construction
  line L55 (45.9, 68.723) -> (10.9392, 144.6427) projected
  line L56 (55.8, 124) -> (85.8, 124) projected
  line L57 (85.8, 74) -> (55.8, 74) projected
  line L58 (55.8, 84) -> (85.8, 84) projected
  arc A26 (-2, -40.8) -> (1, -43.8) centre (1, -40.8) ccw projected
  line L59 (1, -43.8) -> (-2, -43.8) projected
  arc A27 (1, 152) -> (-2, 149) centre (1, 149) ccw projected
  line L60 (-2, 152) -> (1, 152) projected
  point P0 (0, -41.8)
  point P1 (49.923, -2.077)
  point P2 (49.923, 9)
  constraints: 24 end point, 6 parallel, 4 horizontal alignment, 3 horizontal, 3 perpendicular, 2 coincident, 2 vertical alignment
sketch "Sketch37" plane through (0, 41.8, 8) normal (0, 0, 1) x (1, 0, 0)
  point P0 (0, -41.8)
  point P1 (50.9148, -1.0555)
  point P2 (50.9598, 9.0215)
hole "Hole9" at (50.9148, 40.7445, 8) at (50.9598, 50.8215, 8) direction (0, 0, -1) diameter 2.8 depth 12 tip angle 118 counterbore diameter 6 counterbore depth 2.5
sketch "Sketch38" plane through (-2, 75.8, 0) normal (0, 1, 0) x (1, 0, 0)
  arc A0 (84.2577, 17.5746) -> (61.3842, 17.5746) centre (72.821, 16.921) ccw
  ellipse E0 centre (72.821, 16.921) end of major axis (72.516, 16.921) minor radius 0.2753 (72.821, 16.6457) -> (72.821, 17.1962) ccw
  circle A1 centre (72.821, 16.921) radius 0.2753
  arc A2 (72.821, 17.1962) -> (72.821, 16.6457) centre (72.821, 16.921) ccw
  ellipse E1 centre (74.7289, 16.921) end of major axis (74.4239, 16.921) minor radius 0.2753 (74.4284, 16.8738) -> (74.7502, 17.1956) ccw
  point P0 (2, 0)
  constraints: 4 point on circle, 3 centre point, 22 other
sketch "Sketch39" plane through (95.8, 165.8, -16.921) normal (0, 0, -1) x (-1, 0, 0)
  line L0 (2.0001, 23.923) -> (2.0001, -13.923) projected
  line L1 (0, 15) -> (7.958, 15) projected
  line L2 (0, 15) -> (0, 0) projected
  line L3 (7.958, 0) -> (0, 0) projected
  line L4 (7.958, 15) -> (7.958, 0) projected
  line L5 (7.958, -50) -> (0, -50) projected
  line L6 (7.958, -50) -> (7.958, -40) projected
  line L7 (0, -40) -> (7.958, -40) projected
  line L8 (0, -50) -> (0, -40) projected
  line L9 (0, -90) -> (7.958, -90) projected
  line L10 (0, -90) -> (0, -105) projected
  line L11 (7.958, -105) -> (0, -105) projected
  line L12 (7.958, -90) -> (7.958, -105) projected
  line L13 (42, -90) -> (48, -90) projected
  line L14 (42, -90) -> (42, -105) projected
  line L15 (48, -105) -> (42, -105) projected
  line L16 (48, -50) -> (42, -50) projected
  line L17 (42, -40) -> (48, -40) projected
  line L18 (42, -50) -> (42, -40) projected
  line L19 (42, 15) -> (48, 15) projected
  line L20 (42, 15) -> (42, 0) projected
  line L21 (48, 0) -> (42, 0) projected
  line L22 (48, 15) -> (48, 0) projected
  line L23 (48, -50) -> (48, -40) projected
  line L24 (48, -90) -> (48, -105) projected
  point P0 (95.8, -165.8)
  point P1 (3.979, 7.5)
  point P2 (3.979, -45)
  point P3 (3.979, -97.5)
  point P4 (45, -97.5)
  point P5 (45, -45)
  point P6 (45, 7.5)
hole "Hole10" at (91.821, 173.3, -16.921) at (91.821, 120.8, -16.921) at (91.821, 68.3, -16.921) at (50.8, 68.3, -16.9209) at (50.8, 120.8, -16.9209) at (50.8, 173.3, -16.9209) direction (0, 0, 1) diameter 2.9 end through all counterbore diameter 7 counterbore depth 4
ref_plane "Work Plane9" through (54.144, 78.6902, -18.6271) normal (0.4305, -0.9026, 0) x (0.9026, 0.4305, 0)
sketch "Sketch40" plane through (54.144, 78.6902, -18.6271) normal (0.4305, -0.9026, 0) x (0.9026, 0.4305, 0)
  arc A0 (0, 0) -> (-19.3526, 0) centre (-9.6763, 1.7062) ccw projected
  circle A1 centre (-9.6763, 1.7062) radius 6
  point P0 (-82.7466, 18.6271)
  dimension "d252" = 12
  constraints: 1 centre point, 1 coincident
  measures "d252" diameter of A1
extrude "Extrusion23" cut sketch "Sketch40" along normal mid plane 100
hole "Hole11" at (22.6677, 141.1363, 0) at (7.9556, 134.119, 0) at (33.6761, 99.1258, 0) direction (0, 0, 1) diameter 2.8 end through all counterbore diameter 6 counterbore depth 6.5
sketch "Sketch41" plane through (0, 41.8, 0) normal (0, 0, -1) x (-1, 0, 0)
  line L0 (-8.0604, 76.304) -> (12.7031, 119.8357) projected
  line L1 (21.4433, 131.7452) -> (-28.6669, 26.687)
  line L2 (-28.6669, 26.687) -> (-60.8287, 42.0274)
  line L3 (-60.8287, 42.0274) -> (-10.7185, 147.0856)
  line L4 (-10.7185, 147.0856) -> (21.4433, 131.7452)
  point P0 (0, -41.8)
  constraints: 8 end point, 2 parallel, 1 perpendicular
extrude "Extrusion24" cut sketch "Sketch41" against normal blind 4
sketch "Sketch43" plane through (0, 41.8, 0) normal (0, 0, -1) x (-1, 0, 0)
  circle A0 centre (-1, 49) radius 1.6 projected
  circle A1 centre (-41, -41) radius 1.6 projected
  circle A2 centre (-1, -40.8) radius 1.6 projected
  circle A3 centre (-1, -1) radius 1.6 projected
  circle A4 centre (-1, 9) radius 1.6 projected
  circle A5 centre (-1, 59) radius 1.6 projected
  circle A6 centre (-41, 9) radius 1.6 projected
  circle A7 centre (-41, -1) radius 1.6 projected
  line L0 (-38.4, -3.5) -> (-3.4, -3.5) projected
  line L1 (-3.4, -3.5) -> (-3.4, -38.5) projected
  line L2 (-3.4, -38.5) -> (-38.4, -38.5) projected
  line L3 (-38.4, -38.5) -> (-38.4, -3.5) projected
  line L4 (-38.4, 31.3294) -> (-42.9417, 33.4957) projected
  line L5 (-42.9417, 33.4957) -> (-42.9417, -45.8) projected
  line L6 (-42.9417, -45.8) -> (2, -45.8) projected
  arc A8 (2, -45.8) -> (4, -43.8) centre (2, -43.8) ccw projected
  line L7 (4, -43.8) -> (4, 95.1746) projected
  line L8 (4, 95.1746) -> (-19.3011, 46.3229) projected
  line L9 (-19.3011, 46.3229) -> (-3.4, 46.3229) projected
  line L10 (-3.4, 46.3229) -> (-3.4, 11.3229) projected
  line L11 (-3.4, 11.3229) -> (-38.4, 11.3229) projected
  line L12 (-38.4, 11.3229) -> (-38.4, 31.3294) projected
  line L13 (-9.0689, 56.7246) -> (-3.3295, 68.7575)
  line L14 (-3.3295, 68.7575) -> (-5.8525, 69.9609)
  line L15 (-5.8525, 69.9609) -> (-11.5918, 57.928)
  line L16 (-11.5918, 57.928) -> (-9.0689, 56.7246)
  line L17 (4, 95.1746) -> (-19.3011, 46.3229) projected
  point P0 (0, -41.8)
  constraints: 8 end point, 3 parallel, 1 perpendicular
extrude "Extrusion26" cut sketch "Sketch43" against normal through all contours L16 L15 L14 L13
equation "\"d38\" = d37"
equation "\"d39\" = d37"
equation "\"d40\" = d39"
equation "\"d41\" = d37"
equation "\"d42\" = d41"
equation "\"d43\" = d37"
equation "\"d44\" = d43"
body "Solid1"
